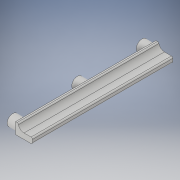
# Autodesk Inventor part: 19 bakjes legger
Saved by Autodesk Inventor 2019 (Build 230136000, 136)
## iProperties
Created: 2020-11-24
Part Number: 19 bakjes legger
Material: Generic
Document SubType Name: Modeling
Designer: Stefan
Density: 1 g/cm^3
Appearance: Default
Author: Stefan
Autodesk Inventor part; units mm, degrees
ref_plane "YZ Plane" through (0, 0, 0) normal (1, 0, 0) x (0, 1, 0)
ref_plane "XZ Plane" through (0, 0, 0) normal (0, 1, 0) x (-1, 0, 0)
ref_plane "XY Plane" through (0, 0, 0) normal (0, 0, 1) x (1, 0, 0)
sketch "Sketch1" plane through (0, 0, 0) normal (0, 0, 1) x (1, 0, 0)
  line L0 (-0.5, -2) -> (0.5, -2)
  line L1 (0.5, 0) -> (0.5, 2)
  line L2 (0.5, 2) -> (-0.5, 2)
  line L3 (-0.5, 2) -> (-0.5, -2)
  line L4 (-0.5, -2) -> (0.5, 2) construction
  line L5 (0.5, -2) -> (-0.5, 2) construction
  line L6 (0.5, -2) -> (5.5, -2)
  line L7 (5.5, -2) -> (5.5, 0)
  line L8 (5.5, 0) -> (0.5, 0)
  point P0 (0, 0)
  dimension "d0" = 1
  dimension "d1" = 4
  dimension "d2" = 5
  dimension "d3" = 14.036
  dimension "d4" = 2
  constraints: 18 end point, 3 parallel, 2 horizontal, 2 midpoint, 2 perpendicular
  measures "d0" distance of L2.end L1.end
  measures "d1" distance of L1.end L0.end
  measures "d2" distance of L0.end L6.end
  measures "d3" angle of L7 L4
  measures "d4" distance between parallel lines of L8 L2
extrude "Extrusion1" add sketch "Sketch1" along normal blind 50
fillet "Fillet1" radius 2 1 edges at (0.5, 0, 25)
fillet "Fillet2" radius 0.5 4 edges at (0.5, 1.9995, 25) (0.5, 2, 25) (5.5, -2, 25) (5.5, 0, 25)
sketch "Sketch2" plane through (-0.5, -2, 0) normal (-1, 0, 0) x (0, 0, 1)
  line L0 (50, 2) -> (0, 2) projected
  circle A0 centre (2, 2) radius 2
  line L1 (0, 4) -> (50, 4) projected
  line L2 (50, 4) -> (50, 0) projected
  circle A1 centre (48, 2) radius 2
  circle A2 centre (25, 2) radius 2
  dimension "d9" = 2
  dimension "d11" = 4
  dimension "d12" = 2
  dimension "d13" = 0
  dimension "d14" = 4
  dimension "d15" = 0
  dimension "d16" = 23
  constraints: 3 centre point, 1 point on line, 1 tangent
  measures "d9" distance of A0.centre L0.end
  measures "d11" diameter of A1
  measures "d12" distance from line of L2 A1.centre
  measures "d13" vertical distance of A0.centre A1.centre
  measures "d14" diameter of A2
  measures "d15" vertical distance of A0.centre A2.centre
  measures "d16" distance of A0.centre A2.centre
extrude "Extrusion2" add sketch "Sketch2" along normal blind 3 contours A0 L0 | L0 A0 | A2 L0 | L0 A2 | A1 L0 | L0 A1
body "Solid1"
